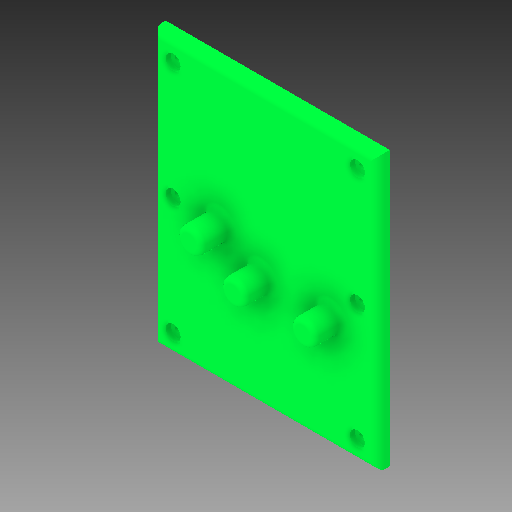
# Autodesk Inventor part: solar_panel_back_lid
Saved by Autodesk Inventor 2018 (Build 220112000, 112)
## iProperties
Created: 2019-04-02
Part Number: solar_panel_back_lid
Material: Generic
Document SubType Name: Modeling
Designer: ZEUSLAP
Density: 1 g/cm^3
Appearance: Default
Mass: 45.5142 g
Surface Area: 234.049 cm^2
Volume: 45.5142 cm^3
Author: ZEUSLAP
## iProperties of the stored document solar_panel_back_lid_3DPrint.ipt
Created: 2019-04-13
Part Number: solar_panel_back_lid_3DPrint
Material: Generic
Document SubType Name: Modeling
Designer: ZEUSLAP
Density: 1 g/cm^3
Appearance: Default
Author: ZEUSLAP
Autodesk Inventor part; units mm, degrees
ref_plane "YZ Plane" through (0, 0, 0) normal (1, 0, 0) x (0, 1, 0)
ref_plane "XZ Plane" through (0, 0, 0) normal (0, 1, 0) x (-1, 0, 0)
ref_plane "XY Plane" through (0, 0, 0) normal (0, 0, 1) x (1, 0, 0)
sketch "Sketch1" plane through (0, 0, 0) normal (0, 0, 1) x (1, 0, 0)
  line L0 (45, -55) -> (-45, -55)
  line L1 (-45, -55) -> (-45, 55)
  line L2 (-45, 55) -> (45, 55)
  line L3 (45, 55) -> (45, -55)
  line L4 (45, -55) -> (-45, 55) construction
  line L5 (-45, -55) -> (45, 55) construction
  circle A0 centre (-37, 157) radius 0.75 projected
  circle A1 centre (37, 157) radius 0.75 projected
  circle A2 centre (37, 204) radius 0.75 projected
  circle A3 centre (-37, 204) radius 0.75 projected
  circle A4 centre (-37, 251) radius 0.75 projected
  circle A5 centre (37, 251) radius 0.75 projected
  point P0 (0, 0)
  dimension "d6" = 90
  dimension "d7" = 110
  constraints: 12 end point, 2 midpoint, 2 parallel, 1 horizontal, 1 perpendicular
  measures "d6" distance of L1.end L2.end
  measures "d7" distance of L0.end L1.end
extrude "1-backlid" add sketch "Sketch1" along normal blind 5 contours L0 L1 L2 L3
fillet "2-fillet_backlid" radius 3 4 edges at (0, 55, 5) (45, 0, 5) (-45, 0, 5) (0, -55, 5)
sketch "Sketch11" plane through (0, 0, 5) normal (0, 0, 1) x (1, 0, 0)
  circle A0 centre (37, 0) radius 3
  circle A1 centre (-37, 0) radius 3
  circle A2 centre (37, 47) radius 3
  circle A3 centre (-37, 47) radius 3
  circle A4 centre (-37, -47) radius 3
  circle A5 centre (37, -47) radius 3
  point P0 (0, 0)
  dimension "d58" = 6
  dimension "d59" = 6
  dimension "d60" = 6
  dimension "d61" = 6
  dimension "d62" = 6
  constraints: 6 centre point
  measures "d58" diameter of A1
  measures "d59" diameter of A3
  measures "d60" diameter of A2
  measures "d61" diameter of A0
  measures "d62" diameter of A5
sketch "Sketch10" plane through (0, 0, 5) normal (0, 0, 1) x (1, 0, 0)
  circle A0 centre (-37, -47) radius 1.25
  circle A1 centre (-37, 0) radius 1.25
  circle A2 centre (-37, 47) radius 1.25
  circle A3 centre (37, 47) radius 1.25
  circle A4 centre (37, 0) radius 1.25
  circle A5 centre (37, -47) radius 1.25
  line L0 (37, -47) -> (-56.3107, -47) construction
  line L1 (-37, 0) -> (-37, -58.4435) construction
  point P0 (0, 0)
  point P1 (-37, -47)
  dimension "d52" = 2.5
  dimension "d53" = 2.5
  dimension "d54" = 2.5
  dimension "d55" = 2.5
  dimension "d56" = 2.5
  dimension "d67" = 2.5
  constraints: 6 centre point, 4 end point, 2 point on line, 1 coincident, 1 horizontal, 1 vertical
  measures "d52" diameter of A1
  measures "d53" diameter of A2
  measures "d54" diameter of A3
  measures "d55" diameter of A4
  measures "d56" diameter of A5
  measures "d67" diameter of A0
extrude "3-screw-head_slots" cut sketch "Sketch11" against normal blind 2
extrude "4-screw_holes" cut sketch "Sketch10" against normal up to surface (5 mm away)
sketch "Sketch4" plane through (0, 0, 0) normal (0, 0, -1) x (-1, 0, 0)
  line L0 (8, -38.25) -> (30, -38.25)
  line L1 (30, -38.25) -> (30, 38.25)
  line L2 (30, 38.25) -> (8, 38.25)
  line L3 (8, 38.25) -> (8, -38.25)
  line L4 (45, -55) -> (-45, -55) construction
  line L5 (0, -55) -> (0, 55) construction
  line L6 (45, 55) -> (-45, 55) construction
  line L7 (0, 0) -> (45, 0) construction
  line L8 (45, 55) -> (45, -55) construction
  point P0 (7.7433, 38.25)
  point P1 (29.7433, -38.25)
  dimension "d68" = 76.5
  dimension "d69" = 22
  dimension "d70" = 8
  dimension "d71" = 38.25
  constraints: 12 end point, 4 midpoint, 2 parallel, 1 horizontal, 1 perpendicular
  measures "d68" distance of L2.end L0.start
  measures "d69" distance of L0.start L0.end
  measures "d70" distance between parallel lines of L5 L3
  measures "d71" distance between parallel lines of L7 L0
extrude "5-battery_holder_slot" cut sketch "Sketch4" against normal blind 2.5
sketch "Sketch5" plane through (0, 0, 0) normal (0, 0, -1) x (-1, 0, 0)
  line L0 (-1.3443, 21) -> (-22.3443, 21)
  line L1 (-22.3443, 21) -> (-22.3443, -21)
  line L2 (-22.3443, -21) -> (-1.3443, -21)
  line L3 (-1.3443, -21) -> (-1.3443, 21)
  line L4 (-1.3443, -21) -> (-22.3443, 21) construction
  line L5 (-1.3443, 21) -> (-22.3443, -21) construction
  point P0 (0, 0)
  point P1 (-11.8443, 0)
  point P2 (-62.3541, 0)
  point P3 (-62.3541, 0)
  dimension "d27" = 21
  dimension "d28" = 42
  constraints: 12 end point, 2 parallel, 1 horizontal, 1 midpoint, 1 perpendicular
  measures "d27" distance of L2.end L1.end
  measures "d28" distance of L1.end L1.start
extrude "6-solar_charger_slot" cut sketch "Sketch5" against normal blind 1.5
sketch "Sketch13" plane through (0, 0, 2.5) normal (0, 0, -1) x (-1, 0, 0)
  circle A0 centre (18.245, 0) radius 5
  point P0 (0, 0)
  dimension "d77" = 10
  constraints: 1 centre point
  measures "d77" diameter of A0
extrude "7-for_battery_holder_screw" add sketch "Sketch13" against normal blind 15
sketch "Sketch8" plane through (0, 0, 1.5) normal (0, 0, -1) x (-1, 0, 0)
  line L0 (-1.3443, -21) -> (-22.3443, -21) construction
  line L1 (-1.3443, -21) -> (-1.3443, -10) construction
  line L2 (-1.3443, -10) -> (1.6557, -10) construction
  line L3 (-22.3443, -21) -> (-22.3443, 21) construction
  line L4 (-22.3443, -10) -> (-26.3443, -10) construction
  circle A0 centre (-26.3443, -10) radius 5
  circle A1 centre (1.6557, -10) radius 5
  point P0 (0, 0)
  dimension "d37" = 11
  dimension "d38" = 3
  dimension "d39" = 4
  dimension "d40" = 10
  dimension "d41" = 10
  dimension "d82" = 28
  constraints: 6 end point, 2 centre point, 2 coincident, 1 horizontal, 1 perpendicular, 1 point on line, 1 vertical
  measures "d37" distance of L0.start L1.end
  measures "d38" distance of L1.end L2.end
  measures "d39" distance of L4.start L4.end
  measures "d40" diameter of A0
  measures "d41" diameter of A1
  measures "d82" distance of L2.end L4.end
extrude "8-for_solar_charger_screws" add sketch "Sketch8" against normal blind 15
sketch "Sketch9" plane through (0, 0, 1.5) normal (0, 0, -1) x (-1, 0, 0)
  circle A0 centre (-26.3443, -10) radius 5 projected
  circle A1 centre (1.6557, -10) radius 5 projected
  circle A2 centre (1.6557, -10) radius 0.75
  circle A3 centre (-26.3443, -10) radius 0.75
  point P0 (0, 0)
  dimension "d44" = 1.5
  dimension "d45" = 1.5
  constraints: 2 centre point, 2 coincident
  measures "d44" diameter of A2
  measures "d45" diameter of A3
extrude "9-holes_solar_charger" cut sketch "Sketch9" against normal blind 12 and the other way blind 6 contours A2 | A3
sketch "Sketch12" plane through (0, 0, 0) normal (0, 0, -1) x (-1, 0, 0)
  circle A0 centre (18.245, 0) radius 0.75
  point P0 (0, 0)
  dimension "d81" = 1.5
  constraints: 1 centre point, 1 coincident
  measures "d81" diameter of A0
extrude "10-holes_battery_holder" cut sketch "Sketch12" against normal blind 14
fillet "11-fillet" radius 2 6 edges at (-13.245, 0, 17.5) (3.3443, -10, 16.5) (31.3443, -10, 16.5) (31.3443, -10, 5) (3.3443, -10, 5) (-13.245, 0, 5)
body "Solid4"
